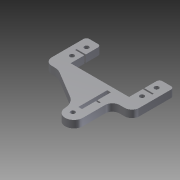
# Autodesk Inventor part: braket atas
Saved by Autodesk Inventor 2012 (Build 160160000, 160)
## iProperties
Created: 2013-12-07
Part Number: braket atas
Material: Default
Document SubType Name: Modeling
Designer: Irwan Haryanto
Density: 1 g/cm^3
Author: Irwan Haryanto
Autodesk Inventor part; units mm, degrees
ref_plane "YZ Plane" through (0, 0, 0) normal (1, 0, 0) x (0, 1, 0)
ref_plane "XZ Plane" through (0, 0, 0) normal (0, 1, 0) x (-1, 0, 0)
ref_plane "XY Plane" through (0, 0, 0) normal (0, 0, 1) x (1, 0, 0)
sketch "Sketch1" plane through (0, 0, 0) normal (0, 0, 1) x (1, 0, 0)
  line L0 (28.55, -23.3) -> (28.55, -3.5)
  line L1 (28.55, -23.3) -> (28.55, -3.5)
  line L2 (31.05, -23.3) -> (31.05, -13.9)
  line L3 (31.05, -23.3) -> (28.55, -23.3)
  line L4 (28.55, -3.5) -> (29.8, -3.5)
  line L5 (28.55, -3.5) -> (31.05, -3.5)
  line L6 (29.8, -3.5) -> (31.05, -3.5)
  line L7 (31.05, -3.5) -> (31.05, -12.9)
  line L8 (31.05, -12.9) -> (31.05, -3.5)
  line L9 (31.05, -13.9) -> (33.55, -13.9)
  line L10 (0, 0) -> (40, 0)
  line L11 (0, 0) -> (39.7, 0)
  line L12 (19.695, -20.087) -> (1.9251, -9.4251)
  line L13 (1.9251, -9.4251) -> (19.695, -20.087)
  line L14 (40, 9.4) -> (46.2, 9.4)
  line L15 (46.54, 9.4) -> (40, 9.4)
  line L16 (46.54, 9.9) -> (46.54, 9.4)
  line L17 (46.2, 10.4) -> (40, 10.4)
  line L18 (46.54, 9.9) -> (46.54, 10.4)
  line L19 (50, 18.8) -> (50, 0)
  line L20 (40, 10.4) -> (40, 18.8)
  line L21 (46.54, 10.4) -> (40, 10.4)
  line L22 (40, 0) -> (40, 9.4)
  line L23 (50, -3) -> (50, 0)
  arc A0 (-8, 20.8) -> (-10, 18.8) centre (-8, 18.8) ccw
  arc A1 (-8, 20.8) -> (-10, 18.8) centre (-8, 18.8) ccw
  line L24 (-2, 20.8) -> (-8, 20.8)
  line L25 (-8, 20.8) -> (-2, 20.8)
  arc A2 (0, 18.8) -> (-2, 20.8) centre (-2, 18.8) ccw
  arc A3 (0, 18.8) -> (-2, 20.8) centre (-2, 18.8) ccw
  arc A4 (24.55, -28.6619) -> (19.695, -20.087) centre (14.55, -28.6619) ccw
  arc A5 (24.55, -28.6619) -> (19.695, -20.087) centre (14.55, -28.6619) ccw
  line L26 (24.55, -28.3) -> (24.55, -28.6619)
  line L27 (24.55, -28.6619) -> (24.55, -28.3)
  arc A6 (42, 20.8) -> (40, 18.8) centre (42, 18.8) ccw
  line L28 (41.7, 20.8) -> (47.7, 20.8)
  line L29 (42, 20.8) -> (48, 20.8)
  arc A7 (47.85, 20.7944) -> (47.7, 20.8) centre (47.7, 18.8) ccw
  arc A8 (50, 18.8) -> (48, 20.8) centre (48, 18.8) ccw
  arc A9 (24.55, -28.3) -> (36.55, -28.3) centre (30.55, -28.3) ccw
  line L30 (29.8, -23.3) -> (29.8, -28.3)
  line L31 (33.55, -13.9) -> (33.55, -12.9)
  line L32 (33.55, -12.9) -> (31.05, -12.9)
  line L33 (36.55, -13) -> (36.55, -14.9)
  line L34 (31.05, -23.3) -> (28.55, -23.3)
  line L35 (31.05, -13.9) -> (31.05, -23.3)
  line L36 (33.55, -13.9) -> (31.05, -13.9)
  line L37 (31.05, -12.9) -> (33.55, -12.9)
  line L38 (33.55, -12.9) -> (33.55, -13.9)
  line L39 (36.55, -14.9) -> (36.55, -28.3)
  line L40 (36.55, -13) -> (36.55, -28.3)
  arc A10 (24.55, -28.3) -> (36.55, -28.3) centre (30.55, -28.3) ccw
  arc A11 (-10, -3) -> (-5, -8) centre (-5, -3) ccw
  line L41 (-3.2198, -8) -> (-5, -8)
  arc A12 (1.9251, -9.4251) -> (-3.2198, -8) centre (-3.2198, -18) ccw
  arc A13 (1.9251, -9.4251) -> (-3.2198, -8) centre (-3.2198, -18) ccw
  line L42 (-3.2198, -8) -> (-5, -8)
  arc A14 (-10, -3) -> (-5, -8) centre (-5, -3) ccw
  line L43 (41.55, -8) -> (45, -8)
  arc A15 (45, -8) -> (50, -3) centre (45, -3) ccw
  arc A16 (41.55, -8) -> (36.55, -13) centre (41.55, -13) ccw
  line L44 (44.7, -8) -> (41.55, -8)
  arc A17 (41.55, -8) -> (36.55, -13) centre (41.55, -13) ccw
  line L45 (0, 18.8) -> (0, 10.4)
  line L46 (0, 18.8) -> (0, 10.4)
  line L47 (-6.35, 9.4) -> (0, 9.4)
  line L48 (-6.35, 10.4) -> (0, 10.4)
  line L49 (0, 10.4) -> (-6.5, 10.4)
  line L50 (-6.5, 9.4) -> (0, 9.4)
  line L51 (0, 9.4) -> (0, 0)
  line L52 (0, 9.4) -> (0, 0)
  line L53 (-6.35, 9.9) -> (-6.35, 9.4)
  line L54 (-6.35, 9.9) -> (-6.35, 10.4)
  line L55 (-6.5, 10.4) -> (-6.5, 9.4)
  line L56 (-10, 18.8) -> (-10, 0)
  line L57 (-10, -3) -> (-10, 18.8)
  line L58 (-10, 0) -> (-10, -3)
  arc A18 (44.7, -8) -> (44.85, -7.9977) centre (44.7, -3) ccw
  point P0 (-10, 20.8)
  point P1 (0, 20.8)
  dimension "d59" = 1.25
  dimension "d60" = 2.5
  dimension "d61" = 19.8
  dimension "d62" = 5
  dimension "d63" = 9.4
  dimension "d64" = 2.5
  dimension "d65" = 1
  dimension "d66" = 1
  dimension "d67" = 1
  dimension "d68" = 5
  dimension "d69" = 10
  dimension "d70" = 10
  dimension "d71" = 2
  dimension "d81" = 40
  dimension "d82" = 40
  dimension "d83" = 10
  dimension "d84" = 10
  dimension "d88" = 6.75
  constraints: 118 end point, 40 point on circle, 19 centre point, 15 tangent, 6 equal radius, 4 point on line, 1 midpoint, 1 perpendicular
  measures "d59" distance of L4.end L6.end
  measures "d60" distance of L2.start L0.start
  measures "d61" distance of L0.start L0.end
  measures "d62" distance of L30.start L30.end
  measures "d63" distance of L2.start L2.end
  measures "d64" distance of L2.end L9.end
  measures "d65" distance of L9.end L31.end
  measures "d66" distance of L15.start L18.end
  measures "d67" distance between parallel lines of L47 L48
  measures "d68" radius of A15
  measures "d69" radius of A12
  measures "d70" distance of point (0, 20.8) point (-10, 20.8)
  measures "d71" radius of A2
  measures "d81" distance between parallel lines of L20 L46
  measures "d82" distance between parallel lines of L22 L51
  measures "d83" distance between parallel lines of L19 L20
  measures "d84" distance between parallel lines of L19 L22
  measures "d88" distance from line of L39 L30.end
extrude "Extrusion1" add sketch "Sketch1" along normal blind 5
sketch "Sketch3" plane through (0, 0, 5) normal (0, 0, 1) x (1, 0, 0)
  line L0 (28.55, -23.3) -> (28.55, -3.5)
  line L1 (28.55, -23.3) -> (28.55, -3.5)
  line L2 (31.05, -23.3) -> (31.05, -13.9)
  line L3 (31.05, -23.3) -> (28.55, -23.3)
  line L4 (28.55, -3.5) -> (29.8, -3.5)
  line L5 (28.55, -3.5) -> (31.05, -3.5)
  line L6 (29.8, -3.5) -> (31.05, -3.5)
  line L7 (31.05, -3.5) -> (31.05, -12.9)
  line L8 (31.05, -12.9) -> (31.05, -3.5)
  line L9 (31.05, -13.9) -> (33.55, -13.9)
  line L10 (0, 0) -> (40, 0)
  line L11 (0, 0) -> (39.7, 0)
  line L12 (19.695, -20.087) -> (1.9251, -9.4251)
  line L13 (1.9251, -9.4251) -> (19.695, -20.087)
  circle A0 centre (44, 4.9) radius 1.5
  line L14 (40, 9.4) -> (46.2, 9.4)
  line L15 (46.54, 9.4) -> (40, 9.4)
  line L16 (46.54, 9.9) -> (46.54, 9.4)
  line L17 (46.2, 10.4) -> (40, 10.4)
  line L18 (46.54, 9.9) -> (46.54, 10.4)
  line L19 (50, 18.8) -> (50, 0)
  circle A1 centre (44, 14.9) radius 1.5
  line L20 (40, 10.4) -> (40, 18.8)
  line L21 (46.54, 10.4) -> (40, 10.4)
  line L22 (40, 0) -> (40, 9.4)
  line L23 (50, -3) -> (50, 0)
  arc A2 (-8, 20.8) -> (-10, 18.8) centre (-8, 18.8) ccw
  arc A3 (-8, 20.8) -> (-10, 18.8) centre (-8, 18.8) ccw
  line L24 (-2, 20.8) -> (-8, 20.8)
  line L25 (-8, 20.8) -> (-2, 20.8)
  arc A4 (0, 18.8) -> (-2, 20.8) centre (-2, 18.8) ccw
  arc A5 (0, 18.8) -> (-2, 20.8) centre (-2, 18.8) ccw
  arc A6 (24.55, -28.6619) -> (19.695, -20.087) centre (14.55, -28.6619) ccw
  arc A7 (24.55, -28.6619) -> (19.695, -20.087) centre (14.55, -28.6619) ccw
  line L26 (24.55, -28.3) -> (24.55, -28.6619)
  line L27 (24.55, -28.6619) -> (24.55, -28.3)
  arc A8 (42, 20.8) -> (40, 18.8) centre (42, 18.8) ccw
  line L28 (41.7, 20.8) -> (47.7, 20.8)
  line L29 (42, 20.8) -> (48, 20.8)
  arc A9 (47.85, 20.7944) -> (47.7, 20.8) centre (47.7, 18.8) ccw
  arc A10 (50, 18.8) -> (48, 20.8) centre (48, 18.8) ccw
  arc A11 (24.55, -28.3) -> (36.55, -28.3) centre (30.55, -28.3) ccw
  line L30 (29.8, -23.3) -> (29.8, -28.3)
  circle A12 centre (29.8, -28.3) radius 1.5
  line L31 (33.55, -13.9) -> (33.55, -12.9)
  line L32 (33.55, -12.9) -> (31.05, -12.9)
  line L33 (36.55, -13) -> (36.55, -14.9)
  line L34 (31.05, -23.3) -> (28.55, -23.3)
  line L35 (31.05, -13.9) -> (31.05, -23.3)
  line L36 (33.55, -13.9) -> (31.05, -13.9)
  line L37 (31.05, -12.9) -> (33.55, -12.9)
  line L38 (33.55, -12.9) -> (33.55, -13.9)
  line L39 (36.55, -14.9) -> (36.55, -28.3)
  line L40 (36.55, -13) -> (36.55, -28.3)
  arc A13 (24.55, -28.3) -> (36.55, -28.3) centre (30.55, -28.3) ccw
  arc A14 (-10, -3) -> (-5, -8) centre (-5, -3) ccw
  line L41 (-3.2198, -8) -> (-5, -8)
  arc A15 (1.9251, -9.4251) -> (-3.2198, -8) centre (-3.2198, -18) ccw
  arc A16 (1.9251, -9.4251) -> (-3.2198, -8) centre (-3.2198, -18) ccw
  line L42 (-3.2198, -8) -> (-5, -8)
  arc A17 (-10, -3) -> (-5, -8) centre (-5, -3) ccw
  line L43 (41.55, -8) -> (45, -8)
  arc A18 (45, -8) -> (50, -3) centre (45, -3) ccw
  arc A19 (41.55, -8) -> (36.55, -13) centre (41.55, -13) ccw
  line L44 (44.7, -8) -> (41.55, -8)
  arc A20 (41.55, -8) -> (36.55, -13) centre (41.55, -13) ccw
  line L45 (0, 18.8) -> (0, 10.4)
  line L46 (0, 18.8) -> (0, 10.4)
  line L47 (-6.35, 9.4) -> (0, 9.4)
  line L48 (-6.35, 10.4) -> (0, 10.4)
  line L49 (0, 10.4) -> (-6.5, 10.4)
  line L50 (-6.5, 9.4) -> (0, 9.4)
  line L51 (0, 9.4) -> (0, 0)
  line L52 (0, 9.4) -> (0, 0)
  circle A21 centre (-4, 14.9) radius 1.5
  circle A22 centre (-4, 4.9) radius 1.5
  line L53 (-6.35, 9.9) -> (-6.35, 9.4)
  line L54 (-6.35, 9.9) -> (-6.35, 10.4)
  line L55 (-6.5, 10.4) -> (-6.5, 9.4)
  line L56 (-10, 18.8) -> (-10, 0)
  line L57 (-10, -3) -> (-10, 18.8)
  line L58 (-10, 0) -> (-10, -3)
  arc A23 (44.7, -8) -> (44.85, -7.9977) centre (44.7, -3) ccw
  point P0 (-10, 20.8)
  point P1 (0, 20.8)
  dimension "d89" = 1.25
  dimension "d90" = 2.5
  dimension "d91" = 19.8
  dimension "d92" = 5
  dimension "d93" = 9.4
  dimension "d94" = 2.5
  dimension "d95" = 1
  dimension "d96" = 1
  dimension "d97" = 1
  dimension "d98" = 5
  dimension "d99" = 10
  dimension "d100" = 10
  dimension "d101" = 2
  dimension "d102" = 10
  dimension "d103" = 10
  dimension "d104" = 4.5
  dimension "d105" = 4.5
  dimension "d106" = 4.5
  dimension "d107" = 4.5
  dimension "d108" = 4
  dimension "d109" = 48
  dimension "d110" = 48
  dimension "d111" = 40
  dimension "d112" = 40
  dimension "d113" = 10
  dimension "d114" = 10
  dimension "d115" = 4
  dimension "d116" = 4
  dimension "d117" = 4
  dimension "d118" = 6.75
  constraints: 118 end point, 40 point on circle, 24 centre point, 15 tangent, 6 equal radius, 4 coincident, 4 point on line, 1 midpoint, 1 perpendicular
  measures "d89" distance of L4.end L6.end
  measures "d90" distance of L2.start L0.start
  measures "d91" distance of L0.start L0.end
  measures "d92" distance of L30.start L30.end
  measures "d93" distance of L2.start L2.end
  measures "d94" distance of L2.end L9.end
  measures "d95" distance of L9.end L31.end
  measures "d96" distance of L15.start L18.end
  measures "d97" distance between parallel lines of L47 L48
  measures "d98" radius of A18
  measures "d99" radius of A15
  measures "d100" distance of point (0, 20.8) point (-10, 20.8)
  measures "d101" radius of A4
  measures "d102" distance of A22.centre point (-4, 14.9)
  measures "d103" distance of A0.centre A1.centre
  measures "d104" distance from line of L21 A1.centre
  measures "d105" distance from line of A0.centre L15
  measures "d106" distance from line of L48 point (-4, 14.9)
  measures "d107" distance from line of L47 A22.centre
  measures "d108" distance from line of L45 point (-4, 14.9)
  measures "d109" distance of A1.centre point (-4, 14.9)
  measures "d110" distance of A0.centre point (-4, 4.9)
  measures "d111" distance between parallel lines of L20 L46
  measures "d112" distance between parallel lines of L22 L51
  measures "d113" distance between parallel lines of L19 L20
  measures "d114" distance between parallel lines of L19 L22
  measures "d115" distance from line of L22 point (44, 4.9)
  measures "d116" distance from line of L20 A1.centre
  measures "d117" distance from line of L52 A22.centre
  measures "d118" distance from line of L39 L30.end
hole "Hole2" at (-4, 14.9, 5) at (-4, 4.9, 5) at (44, 14.9, 5) at (44, 4.9, 5) at (29.8, -28.3, 5) direction (0, 0, -1) diameter 3 end through all
body "Solid1"
